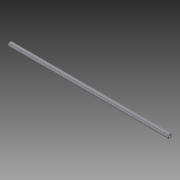
# Autodesk Inventor part: churro_long
Saved by Autodesk Inventor 2015 SP1 (Build 190203100, 203)
## iProperties
Created: 2015-01-13
Part Number: churro_long
Material: Aluminum 6061
Document SubType Name: Modeling
Designer: Jarod
Density: 2.7 g/cm^3
Appearance: Aluminum - Flat
Author: Jarod
Autodesk Inventor part; units mm, degrees
ref_plane "YZ Plane" through (0, 0, 0) normal (1, 0, 0) x (0, 1, 0)
ref_plane "XZ Plane" through (0, 0, 0) normal (0, 1, 0) x (-1, 0, 0)
ref_plane "XY Plane" through (0, 0, 0) normal (0, 0, 1) x (1, 0, 0)
sketch "Sketch1" plane through (0, 0, 0) normal (1, 0, 0) x (0, 1, 0)
  line L0 (6.35, 3.6662) -> (6.35, -3.6662) construction
  line L1 (6.35, -3.6662) -> (0, -7.3323) construction
  line L2 (0, -7.3323) -> (-6.35, -3.6662) construction
  line L3 (-6.35, -3.6662) -> (-6.35, 3.6662) construction
  line L4 (-6.35, 3.6662) -> (0, 7.3323) construction
  line L5 (0, 7.3323) -> (6.35, 3.6662) construction
  line L6 (5.5563, -3.2079) -> (5.5563, 3.2079) construction
  line L7 (5.5563, 3.2079) -> (0, 6.4158) construction
  line L8 (0, 6.4158) -> (-5.5563, 3.2079) construction
  line L9 (-5.5563, 3.2079) -> (-5.5563, -3.2079) construction
  line L10 (-5.5563, -3.2079) -> (0, -6.4158) construction
  line L11 (0, -6.4158) -> (5.5563, -3.2079) construction
  line L12 (6.35, 3.6662) -> (6.35, 1.2849)
  line L13 (6.35, 3.6662) -> (4.2878, 4.8568)
  line L14 (6.35, -3.6662) -> (6.35, -1.2849)
  line L15 (6.35, -3.6662) -> (4.2878, -4.8568)
  line L16 (0, -7.3323) -> (2.0622, -6.1417)
  line L17 (0, -7.3323) -> (-2.0622, -6.1417)
  line L18 (-6.35, -3.6662) -> (-4.2878, -4.8568)
  line L19 (-6.35, -3.6662) -> (-6.35, -1.2849)
  line L20 (-6.35, 3.6662) -> (-6.35, 1.2849)
  line L21 (-6.35, 3.6662) -> (-4.2878, 4.8568)
  line L22 (0, 7.3323) -> (2.0622, 6.1417)
  line L23 (0, 7.3323) -> (-2.0622, 6.1417)
  line L24 (6.35, 1.2849) -> (5.5563, 0.8267)
  line L25 (6.35, 1.2849) -> (7.2665, 1.2849) construction
  line L26 (6.35, -1.2849) -> (5.5563, -0.8267)
  line L27 (6.35, -1.2849) -> (7.2665, -1.2849) construction
  line L28 (5.5563, -0.8267) -> (5.5563, 0.8267)
  line L29 (4.2878, -4.8568) -> (3.494, -4.3985)
  line L30 (4.2878, -4.8568) -> (5.2043, -4.8568) construction
  line L31 (2.0622, -6.1417) -> (2.0622, -5.2252)
  line L32 (2.0622, -6.1417) -> (2.9788, -6.1417) construction
  line L33 (-2.0622, -6.1417) -> (-2.0622, -5.2252)
  line L34 (-2.0622, -6.1417) -> (-1.1457, -6.1417) construction
  line L35 (3.494, -4.3985) -> (2.0622, -5.2252)
  line L36 (-4.2878, -4.8568) -> (-3.494, -4.3985)
  line L37 (-4.2878, -4.8568) -> (-3.3712, -4.8568) construction
  line L38 (-3.494, -4.3985) -> (-2.0622, -5.2252)
  line L39 (-6.35, -1.2849) -> (-5.5563, -0.8267)
  line L40 (-6.35, -1.2849) -> (-5.4335, -1.2849) construction
  line L41 (-6.35, 1.2849) -> (-5.5563, 0.8267)
  line L42 (-6.35, 1.2849) -> (-5.4335, 1.2849) construction
  line L43 (-5.5563, 0.8267) -> (-5.5563, -0.8267)
  line L44 (-4.2878, 4.8568) -> (-3.494, 4.3985)
  line L45 (-4.2878, 4.8568) -> (-3.3712, 4.8568) construction
  line L46 (-2.0622, 6.1417) -> (-2.0622, 5.2252)
  line L47 (-2.0622, 6.1417) -> (-1.1457, 6.1417) construction
  line L48 (-2.0622, 5.2252) -> (-3.494, 4.3985)
  line L49 (2.0622, 6.1417) -> (2.0622, 5.2252)
  line L50 (2.0622, 6.1417) -> (2.9788, 6.1417) construction
  line L51 (4.2878, 4.8568) -> (3.494, 4.3985)
  line L52 (4.2878, 4.8568) -> (5.2043, 4.8568) construction
  line L53 (3.494, 4.3985) -> (2.0622, 5.2252)
  circle A0 centre (0, 0) radius 3.175
  dimension "d0" = 12.7
  dimension "d1" = 12.7
  dimension "d2" = 12.7
  dimension "d3" = 120
  dimension "d4" = 120
  dimension "d5" = 6.35
  dimension "d6" = 6.35
  dimension "d7" = 6.35
  dimension "d11" = 0.7937
  dimension "d12" = 2.3813
  dimension "d13" = 2.3813
  dimension "d14" = 2.3813
  dimension "d15" = 2.3813
  dimension "d16" = 2.3813
  dimension "d17" = 2.3813
  dimension "d18" = 2.3813
  dimension "d19" = 2.3813
  dimension "d20" = 2.3813
  dimension "d21" = 2.3813
  dimension "d22" = 2.3813
  dimension "d23" = 2.3813
  dimension "d24" = 150
  dimension "d25" = 150
  dimension "d26" = 150
  dimension "d27" = 90
  dimension "d28" = 90
  dimension "d29" = 30
  dimension "d30" = 30
  dimension "d31" = 30
  dimension "d32" = 30
  dimension "d33" = 90
  dimension "d34" = 90
  dimension "d35" = 150
  dimension "d36" = 6.35
  constraints: 108 end point, 24 point on line, 12 equal length, 12 horizontal, 6 parallel, 3 collinear, 1 centre point, 1 coincident, 1 vertical, 5 other
  measures "d0" distance between parallel lines of L3 L0
  measures "d1" distance between parallel lines of L4 L1
  measures "d2" distance between parallel lines of L5 L2
  measures "d3" angle of L0 L5
  measures "d4" angle of L1 L0
  measures "d5" distance from line of point (0, 0) L0
  measures "d6" distance from line of point (0, 0) L1
  measures "d7" distance from line of point (0, 0) L5
  measures "d11" distance between parallel lines of L6 L0
  measures "d12" distance of L0.start L12.end
  measures "d13" distance of L0.start L13.end
  measures "d14" distance of L0.end L14.end
  measures "d15" distance of L0.end L15.end
  measures "d16" distance of L1.end L16.end
  measures "d17" distance of L1.end L17.end
  measures "d18" distance of L2.end L18.end
  measures "d19" distance of L2.end L19.end
  measures "d20" distance of L3.end L20.end
  measures "d21" distance of L3.end L21.end
  measures "d22" distance of L4.end L22.end
  measures "d23" distance of L4.end L23.end
  measures "d24" angle of L24 L25
  measures "d25" angle of L27 L26
  measures "d26" angle of L30 L29
  measures "d27" angle of L32 L31
  measures "d28" angle of L34 L33
  measures "d29" angle of L37 L36
  measures "d30" angle of L40 L39
  measures "d31" angle of L41 L42
  measures "d32" angle of L44 L45
  measures "d33" angle of L46 L47
  measures "d34" angle of L49 L50
  measures "d35" angle of L51 L52
  measures "d36" diameter of A0
extrude "Extrusion1" add sketch "Sketch1" along normal blind 546.1
body "Solid1"
